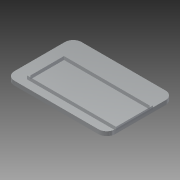
# Autodesk Inventor part: obudowa - budzik v3 plexi
Saved by Autodesk Inventor 2014 (Build 180170000, 170)
## iProperties
Created: 2018-03-05
Part Number: obudowa - budzik v3 plexi
Material: Glass
Document SubType Name: Modeling
Designer: HP820
Density: 1 g/cm^3
Appearance: Clear
Author: HP820
Autodesk Inventor part; units mm, degrees
ref_plane "YZ Plane" through (0, 0, 0) normal (1, 0, 0) x (0, 1, 0)
ref_plane "XZ Plane" through (0, 0, 0) normal (0, 1, 0) x (-1, 0, 0)
ref_plane "XY Plane" through (0, 0, 0) normal (0, 0, 1) x (1, 0, 0)
sketch "Sketch1" plane through (0, 0, 0) normal (0, 0, 1) x (1, 0, 0)
  spline S0 degree 3 poles (-30, -5) (-30, -4.3586) (-29.8694, -3.6802) (-29.3471, -2.4395) (-28.9555, -1.8763) (-28.0866, -1.0236) (-27.5672, -0.665) (-27, -0.4174) knots 1.621626 1.621626 1.621626 1.621626 1.814042 1.814042 2.006457 2.006457 2.182648 2.182648 2.182648 2.182648 projected
  line L0 (-25, 0) -> (25, 0) projected
  spline S1 degree 3 poles (27, -0.4174) (27.5672, -0.665) (28.0866, -1.0236) (28.9555, -1.8763) (29.3471, -2.4395) (29.8694, -3.6802) (30, -4.3586) (30, -5) knots -0.561022 -0.561022 -0.561022 -0.561022 -0.384831 -0.384831 -0.192415 -0.192415 0 0 0 0 projected
  line L1 (30, -5) -> (30, -35) projected
  spline S2 degree 3 poles (30, -35) (30, -35.6414) (29.8694, -36.3198) (29.3471, -37.5605) (28.9555, -38.1237) (28.0866, -38.9764) (27.5672, -39.335) (27, -39.5826) knots 0 0 0 0 0.192415 0.192415 0.384831 0.384831 0.561022 0.561022 0.561022 0.561022 projected
  line L2 (25, -40) -> (-25, -40) projected
  line L3 (-30, -35) -> (-30, -5) projected
  spline S3 degree 3 poles (-27, -39.5826) (-27.5672, -39.335) (-28.0866, -38.9764) (-28.9555, -38.1237) (-29.3471, -37.5605) (-29.8694, -36.3198) (-30, -35.6414) (-30, -35) knots 1.060605 1.060605 1.060605 1.060605 1.236796 1.236796 1.429211 1.429211 1.621626 1.621626 1.621626 1.621626 projected
  arc A0 (-25, 0) -> (-27, -0.4174) centre (-25, -5) ccw projected
  arc A1 (27, -0.4174) -> (25, 0) centre (25, -5) ccw projected
  arc A2 (25, -40) -> (27, -39.5826) centre (25, -35) ccw projected
  arc A3 (-27, -39.5826) -> (-25, -40) centre (-25, -35) ccw projected
  point P0 (0, 0)
extrude "Extrusion1" add sketch "Sketch1" along normal blind 2.5
sketch "Sketch2" plane through (0, 0, 0) normal (0, 0, -1) x (-1, 0, 0)
  line L0 (-25.5, -10) -> (25.5, -10)
  line L1 (25.5, -10) -> (25.5, -30)
  line L2 (25.5, -30) -> (-25.5, -30)
  line L3 (-25.5, -30) -> (-25.5, -10)
  line L4 (-25.5, -10) -> (25.5, -30) construction
  line L5 (25.5, -10) -> (-25.5, -30) construction
  line L6 (-26.5, -9) -> (26.5, -9)
  line L7 (26.5, -9) -> (26.5, -31)
  line L8 (26.5, -31) -> (-26.5, -31)
  line L9 (-26.5, -31) -> (-26.5, -9)
  line L10 (-26.5, -9) -> (26.5, -31) construction
  line L11 (26.5, -9) -> (-26.5, -31) construction
  point P0 (0, 0)
  point P1 (0, -20)
  point P2 (0, -20)
  dimension "d2" = 51
  dimension "d3" = 20
  dimension "d4" = 53
  dimension "d5" = 22
  constraints: 24 end point, 6 midpoint, 4 parallel, 2 horizontal, 2 perpendicular
  measures "d2" distance of L1.end L2.end
  measures "d3" distance of L0.end L1.end
  measures "d4" distance of L7.end L8.end
  measures "d5" distance of L6.end L7.end
extrude "Extrusion2" add sketch "Sketch2" along normal blind 2
body "Solid1"
